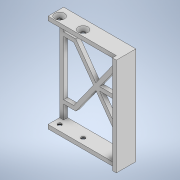
# Autodesk Inventor part: face-1
Saved by Autodesk Inventor 2021 (Build 250183000, 183)
## iProperties
Created: 2024-07-20
Part Number: face-1
Material: Generic
Document SubType Name: Modeling
Designer: Toby
Density: 1 g/cm^3
Appearance: Default
Author: Toby
Autodesk Inventor part; units mm, degrees
ref_plane "YZ Plane" through (0, 0, 0) normal (1, 0, 0) x (0, 1, 0)
ref_plane "XZ Plane" through (0, 0, 0) normal (0, 1, 0) x (-1, 0, 0)
ref_plane "XY Plane" through (0, 0, 0) normal (0, 0, 1) x (1, 0, 0)
sketch "Sketch1" plane through (0, 0, 0) normal (0, 0, 1) x (1, 0, 0)
  line L0 (-45.7037, 34.1852) -> (-8.7037, 34.1852)
  line L1 (-8.7037, 34.1852) -> (-8.7037, -15.8148)
  line L2 (-8.7037, -15.8148) -> (-45.7037, -15.8148)
  line L3 (-45.7037, -15.8148) -> (-45.7037, 34.1852)
  line L4 (-43.7037, 32.1852) -> (-10.7037, 32.1852)
  line L5 (-10.7037, 32.1852) -> (-10.7037, -13.8148)
  line L6 (-10.7037, -13.8148) -> (-43.7037, -13.8148)
  line L7 (-43.7037, -13.8148) -> (-43.7037, 32.1852)
  point P0 (0, 0)
  dimension "d0" = 2
  dimension "d1" = 2
  dimension "d2" = 2
  dimension "d3" = 2
  dimension "d4" = 37
  dimension "d5" = 50
  constraints: 16 end point, 4 parallel, 2 horizontal, 2 perpendicular
  measures "d0" distance between parallel lines of L4 L0
  measures "d1" distance between parallel lines of L2 L6
  measures "d2" distance between parallel lines of L3 L7
  measures "d3" distance between parallel lines of L1 L5
  measures "d4" distance of L0.start L0.end
  measures "d5" distance of L2.end L0.start
extrude "Extrusion1" add sketch "Sketch1" along normal blind 2
sketch "Sketch2" plane through (0, 0, 2) normal (0, 0, 1) x (1, 0, 0)
  line L0 (-43.7037, 32.1852) -> (-10.7037, 32.1852) projected
  line L1 (-10.7037, -13.8148) -> (-43.7037, -13.8148) projected
  line L2 (-43.7037, 32.1852) -> (-10.7037, -13.8148) construction
  line L3 (-44.5162, 31.6023) -> (-11.5162, -14.3977)
  line L4 (-9.8912, -13.2319) -> (-42.8912, 32.7681)
  arc A0 (-42.8912, 32.7681) -> (-44.5162, 31.6023) centre (-43.7037, 32.1852) ccw
  arc A1 (-11.5162, -14.3977) -> (-9.8912, -13.2319) centre (-10.7037, -13.8148) ccw
  line L5 (-10.7037, 32.1852) -> (-10.7037, -13.8148) projected
  line L6 (-10.7037, 32.1852) -> (-43.7037, -13.8148) construction
  line L7 (-11.5162, 32.7681) -> (-44.5162, -13.2319)
  line L8 (-42.8912, -14.3977) -> (-9.8912, 31.6023)
  arc A2 (-9.8912, 31.6023) -> (-11.5162, 32.7681) centre (-10.7037, 32.1852) ccw
  arc A3 (-44.5162, -13.2319) -> (-42.8912, -14.3977) centre (-43.7037, -13.8148) ccw
  point P0 (0, 0)
  point P1 (-27.2037, 9.1852)
  point P2 (-27.2037, 9.1852)
  point P3 (-25.973, 9.1852)
  point P4 (-27.2037, 10.9007)
  point P5 (-28.4344, 9.1852)
  point P6 (-27.2037, 7.4696)
  dimension "d8" = 2
  dimension "d9" = 2
  constraints: 16 end point, 8 point on circle, 8 tangent, 4 centre point, 2 midpoint, 2 parallel
  measures "d8" diameter of A1
  measures "d9" diameter of A3
extrude "Extrusion2" add sketch "Sketch2" against normal blind 2 contours L4 L7 L3 A0 | L7 A2 L8 L5 L0 | L0 L5 L8 L4 L7 | L4 L8 L3 L7 | L4 L5 L1 L3 L8 | L3 L8 A3 L7 | L4 A1 L3 L1 L5
sketch "Sketch3" plane through (0, 0, 2) normal (0, 0, 1) x (1, 0, 0)
  line L0 (-45.7037, 34.1852) -> (-45.7037, -15.8148) projected
  line L1 (-8.7037, -15.8148) -> (-8.7037, 34.1852) projected
  line L2 (-45.7037, 34.1852) -> (-8.7037, 34.1852)
  line L3 (-8.7037, 34.1852) -> (-8.7037, 32.1852)
  line L4 (-8.7037, 32.1852) -> (-45.7037, 32.1852)
  line L5 (-45.7037, 32.1852) -> (-45.7037, 34.1852)
  line L6 (-45.7037, -15.8148) -> (-8.7037, -15.8148)
  line L7 (-8.7037, -15.8148) -> (-8.7037, -13.8148)
  line L8 (-8.7037, -13.8148) -> (-45.7037, -13.8148)
  line L9 (-45.7037, -13.8148) -> (-45.7037, -15.8148)
  line L10 (-42.473, 32.1852) -> (-11.9344, 32.1852) projected
  line L11 (-11.9344, -13.8148) -> (-42.473, -13.8148) projected
  line L12 (-45.7037, -15.8148) -> (-8.7037, -15.8148) projected
  point P0 (0, 0)
  point P1 (-8.7037, 34.1852)
  constraints: 16 end point, 4 parallel, 3 collinear, 3 point on line, 2 horizontal, 2 perpendicular
extrude "Extrusion3" add sketch "Sketch3" along normal blind 6 contours L2 L1 L4 L0 | L8 L1 L6 L0
sketch "Sketch4" plane through (-45.7037, 34.1852, 0) normal (0, 1, 0) x (1, 0, 0)
  line L0 (37, -8) -> (0, -8) projected
  line L1 (0, 0) -> (0, -8) projected
  point P0 (45.7037, 0)
  point P1 (3, -5)
  point P2 (15, -5)
  dimension "d14" = 3
  dimension "d15" = 3
  dimension "d16" = 3
  dimension "d17" = 12
  measures "d14" distance from line of L0 point (3, -5)
  measures "d15" distance from line of L0 point (15, -5)
  measures "d16" distance from line of L1 point (3, -5)
  measures "d17" distance of point (15, -5) point (3, -5)
hole "Hole1" at (-42.7037, 34.1852, 5) at (-30.7037, 34.1852, 5) direction (0, -1, 0) diameter 2 depth 10 tip angle 118 countersink diameter 5 countersink angle 90
sketch "Sketch5" plane through (-45.7037, -15.8148, 0) normal (0, -1, 0) x (1, 0, 0)
  circle A0 centre (15, 5) radius 1 projected
  circle A1 centre (3, 5) radius 1 projected
  point P0 (45.7037, 0)
  constraints: 2 coincident
hole "Hole2" at (-30.7037, -15.8148, 5) at (-42.7037, -15.8148, 5) direction (0, 1, 0) diameter 2 depth 10 tip angle 118 countersink diameter 5 countersink angle 90
sketch "Sketch6" plane through (0, 0, 0) normal (0, 0, -1) x (-1, 0, 0)
  line L0 (11.9344, -13.8148) -> (42.473, -13.8148) projected
  line L1 (43.7037, -12.0993) -> (43.7037, 30.4696) projected
  line L2 (17.7037, -13.8148) -> (43.7037, -13.8148)
  line L3 (43.7037, -13.8148) -> (43.7037, -6.8148)
  line L4 (43.7037, -6.8148) -> (17.7037, -6.8148)
  line L5 (17.7037, -6.8148) -> (17.7037, -13.8148)
  line L6 (17.7037, 32.1852) -> (43.7037, 32.1852)
  line L7 (43.7037, 32.1852) -> (43.7037, 25.1852)
  line L8 (43.7037, 25.1852) -> (17.7037, 25.1852)
  line L9 (17.7037, 25.1852) -> (17.7037, 32.1852)
  line L10 (42.473, 32.1852) -> (11.9344, 32.1852) projected
  line L11 (45.7037, 34.1852) -> (45.7037, -15.8148) projected
  line L12 (8.7037, 34.1852) -> (45.7037, 34.1852) projected
  line L13 (45.7037, -15.8148) -> (8.7037, -15.8148) projected
  point P0 (0, 0)
  dimension "d35" = 28
  dimension "d36" = 28
  dimension "d37" = 9
  dimension "d38" = 9
  constraints: 16 end point, 4 parallel, 3 point on line, 2 horizontal, 2 perpendicular, 1 collinear
  measures "d35" distance between parallel lines of L11 L5
  measures "d36" distance between parallel lines of L11 L9
  measures "d37" distance between parallel lines of L12 L8
  measures "d38" distance between parallel lines of L13 L4
extrude "Extrusion4" cut sketch "Sketch6" against normal blind 2
sketch "Sketch7" plane through (0, 0, 0) normal (0, 0, -1) x (-1, 0, 0)
  line L0 (39.9127, -6.8148) -> (37.4513, -6.8148) projected
  line L1 (43.7037, -13.8148) -> (43.7037, 32.1852) projected
  line L2 (37.4513, -6.8148) -> (43.7037, -6.8148)
  line L3 (43.7037, -6.8148) -> (43.7037, -4.8148)
  line L4 (43.7037, -4.8148) -> (37.4513, -4.8148)
  line L5 (37.4513, -4.8148) -> (37.4513, -6.8148)
  line L6 (37.4513, 25.1852) -> (39.9127, 25.1852) projected
  line L7 (37.4513, 25.1852) -> (43.7037, 25.1852)
  line L8 (43.7037, 25.1852) -> (43.7037, 23.1852)
  line L9 (43.7037, 23.1852) -> (37.4513, 23.1852)
  line L10 (37.4513, 23.1852) -> (37.4513, 25.1852)
  point P0 (0, 0)
  dimension "d41" = 2
  dimension "d42" = 2
  constraints: 16 end point, 4 parallel, 2 horizontal, 2 perpendicular, 2 point on line
  measures "d41" distance of L3.end L2.end
  measures "d42" distance of L7.end L8.end
extrude "Extrusion5" add sketch "Sketch7" against normal blind 2
sketch "Sketch8" plane through (0, 0, 0) normal (0, 0, -1) x (-1, 0, 0)
  line L0 (10.7037, -12.0993) -> (25.973, 9.1852) projected
  line L1 (25.973, 9.1852) -> (10.7037, 9.1852) construction
  line L2 (10.7037, 30.4696) -> (10.7037, -12.0993) projected
  line L3 (25.973, 10.1852) -> (10.7037, 10.1852)
  line L4 (10.7037, 8.1852) -> (25.973, 8.1852)
  arc A0 (25.973, 8.1852) -> (25.973, 10.1852) centre (25.973, 9.1852) ccw
  arc A1 (10.7037, 10.1852) -> (10.7037, 8.1852) centre (10.7037, 9.1852) ccw
  point P0 (0, 0)
  point P1 (18.3383, 9.1852)
  dimension "d45" = 2
  constraints: 8 end point, 4 point on circle, 4 tangent, 2 centre point, 2 midpoint, 1 parallel
  measures "d45" diameter of A1
extrude "Extrusion6" add sketch "Sketch8" against normal blind 2 contours L4 L2 L3 A0 | A1 L2
sketch "Sketch9" plane through (-8.7037, -15.8148, 0) normal (1, 0, 0) x (0, 0, -1)
  line L0 (0, 50) -> (-8, 50) projected
  line L1 (0, 0) -> (-8, 0) projected
  line L2 (0, 50) -> (-10, 50)
  line L3 (-10, 50) -> (-10, 0)
  line L4 (-10, 0) -> (0, 0)
  line L5 (0, 0) -> (0, 50)
  point P0 (0, 15.8148)
  dimension "d48" = 10
  constraints: 8 end point, 2 parallel, 1 horizontal, 1 perpendicular, 1 point on line
  measures "d48" distance between parallel lines of L5 L3
extrude "Extrusion7" add sketch "Sketch9" against normal blind 2
fillet "Fillet1" radius 1 2 edges at (-10.7037, 32.1852, 5) (-10.7037, -13.8148, 5)
body "Solid1"
